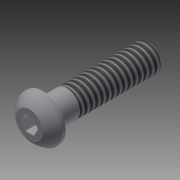
# Autodesk Inventor part: Axle Peg
Saved by Autodesk Inventor 2015 (Build 190159000, 159)
## iProperties
Created: 2018-03-27
Part Number: Axle Peg
Material: Generic
Document SubType Name: Modeling
Designer: Administrator
Density: 1 g/cm^3
Appearance: Default
Mass: 0.993962 g
Surface Area: 7.69141 cm^2
Volume: 0.993962 cm^3
Author: Administrator
Autodesk Inventor part; units mm, degrees
ref_plane "YZ Plane" through (0, 0, 0) normal (1, 0, 0) x (0, 1, 0)
ref_plane "XZ Plane" through (0, 0, 0) normal (0, 1, 0) x (-1, 0, 0)
ref_plane "XY Plane" through (0, 0, 0) normal (0, 0, 1) x (1, 0, 0)
sketch "Sketch1" plane through (0, 0, 0) normal (0, 1, 0) x (-1, 0, 0)
  line L0 (0, 0) -> (3.175, 0)
  line L1 (5.3594, -2.3876) -> (5.3594, -3.175)
  line L2 (5.3594, -3.175) -> (3.175, -3.175)
  line L3 (3.175, -3.175) -> (3.175, -28.575)
  line L4 (3.175, -28.575) -> (0, -28.575)
  line L5 (0, -28.575) -> (0, 0)
  arc A0 (5.3594, -2.3876) -> (3.175, 0) centre (0.0087, -5.0899) ccw
  dimension "d0" = 3.175
  dimension "d1" = 5.3594
  dimension "d2" = 0.7874
  dimension "d3" = 3.175
  dimension "d8" = 3.175
  dimension "d9" = 5.9944
  dimension "d20" = 25.4
  constraints: 12 end point, 3 perpendicular, 2 point on circle, 1 centre point, 1 horizontal, 1 parallel
  measures "d0" distance between parallel lines of L5 L3
  measures "d1" distance from line of L1.end L5
  measures "d2" distance of L1.start L1.end
  measures "d3" distance between parallel lines of L2 L0
  measures "d8" distance of L0.start L0.end
  measures "d9" radius of A0
  measures "d20" distance between parallel lines of L2 L4
revolve "Revolution1" add sketch "Sketch1" angle 360 about axis through (0, 0, -28.575) along (0, 0, 1)
chamfer "Chamfer1" distance 0.762 angle 45 1 edges at (3.175, 0, -28.575)
sketch "Sketch2" plane through (0, 0, 0) normal (0, 0, 1) x (1, 0, 0)
  line L0 (1.9844, 0) -> (0.9922, -1.7185)
  line L1 (0.9922, -1.7185) -> (-0.9922, -1.7185)
  line L2 (-0.9922, -1.7185) -> (-1.9844, 0)
  line L3 (-1.9844, 0) -> (-0.9922, 1.7185)
  line L4 (-0.9922, 1.7185) -> (0.9922, 1.7185)
  line L5 (0.9922, 1.7185) -> (1.9844, 0)
  point P0 (0, 0)
  point P1 (0, 0)
  dimension "d14" = 3.9688
  constraints: 12 end point, 1 coincident, 13 other
  measures "d14" distance of L0.start L2.end
extrude "Extrusion1" cut sketch "Sketch2" against normal blind 2.8194
thread "Thread1" size "1/4-20 UNC" class "2A" standard "ANSI Unified Screw Threads" length 19.05
body "Solid1"
